Autodesk Fusion 360 part; units mm, degrees
(part 2 of 2)
extrude "Extrude27" add sketch "Back" against normal blind 3 separate body contours L0 L1 L2 L3 L6 L7 L8 L15 L16 L17 L20 L21 L22 L23 L24 L26 L29 L30 L31 L33 L34 L35 makes body 2
extrude "Extrude28" add sketch "Bottom" along normal blind 3 separate body contours L0 L1 L2 L3 L7 L8 L9 L11 L12 L13 L17 L19 L20 L23 L25 L26 L30 L31 L33 L34 L36 L37 L38 L39 L40 L44 L45 L47 makes body 3
combine "Combine15" operation cut target body 2 tool bodies 3 keep tools
combine "Combine16" operation cut target body 1 tool bodies 3 keep tools
extrude "Extrude29" add sketch "Right" against normal blind 3 separate body contours L0 L1 L2 L3 L7 L8 L9 L12 L13 L14 makes body 4
combine "Combine17" operation cut target body 4 tool bodies 1 keep tools
extrude "Extrude30" add sketch "Left" along normal blind 3 separate body contours L46 L47 L48 L49 L53 L54 L55 L57 L58 L59 makes body 5
combine "Combine18" operation cut target body 5 tool bodies 1 keep tools
combine "Combine19" operation cut target body 5 tool bodies 2 keep tools
combine "Combine20" operation cut target body 4 tool bodies 2 keep tools
combine "Combine21" operation cut target body 5 tool bodies 3 keep tools
combine "Combine22" operation cut target body 4 tool bodies 3 keep tools
combine "Combine23" operation cut target body 2 tool bodies 3 keep tools
extrude "Extrude31" add sketch "Top" against normal blind 3 separate body makes body 6
combine "Combine24" operation cut target body 6 tool bodies 5 keep tools
combine "Combine25" operation cut target body 6 tool bodies 1 keep tools
combine "Combine26" operation cut target body 6 tool bodies 4 keep tools
combine "Combine27" operation cut target body 6 tool bodies 2 keep tools
extrude "Extrude32" add sketch "BackSupport" along normal blind 3 separate body makes body 7
extrude "Extrude33" add sketch "FrontSupport" along normal blind 3 separate body makes body 8
combine "Combine28" operation cut target body 5 tool bodies 7 keep tools
combine "Combine29" operation cut target body 2 tool bodies 7 keep tools
combine "Combine30" operation cut target body 4 tool bodies 7 keep tools
combine "Combine31" operation cut target body 5 tool bodies 8 keep tools
combine "Combine32" operation cut target body 4 tool bodies 8 keep tools
extrude "Extrude11" [suppressed]
hidden bodies 6
equation "width = 57 mm"
equation "thick = 3 mm"
equation "d31 = -height / 2"
equation "d32 = width"
equation "d33 = length"
equation "d34 = finger"
equation "d35 = thick"
equation "d36 = finger"
equation "d37 = thick"
equation "d38 = finger"
equation "d39 = finger"
equation "d44 = length / 2"
equation "d45 = width"
equation "d46 = height"
equation "d47 = thick"
equation "d48 = finger"
equation "d49 = finger"
equation "height = 51.8 mm"
equation "length = 69 mm"
equation "finger = height / 5"
equation "d60 = -length / 2"
equation "d61 = width"
equation "d62 = height"
equation "d63 = thick"
equation "d64 = finger"
equation "d73 = width / 2"
equation "d74 = length"
equation "d75 = height"
equation "supportHeight = 22 mm + thick"
equation "d82 = -height / 2 + supportHeight"
equation "d83 = width / 2 - thick"
equation "d84 = length / 2 - thick"
equation "d85 = finger"
equation "d86 = backSupportWidth / 2"
equation "d87 = backSupportWidth / 2"
equation "d88 = thick"
equation "d89 = backSupportWidth / 2"
equation "d90 = thick"
equation "d91 = backSupportWidth / 2"
equation "backSupportDepth = 11 mm"
equation "backSupportCutout = 3 mm"
equation "d94 = backSupportWidth"
equation "d95 = backSupportDepth"
equation "d97 = width / 2 - thick - backSupportWidth"
equation "backSupportWidth = 8 mm"
equation "d102 = backSupportCutout"
equation "d103 = width / 2 - thick"
equation "d104 = length / 2 - thick"
equation "d105 = backSupportWidth / 2"
equation "d108 = backSupportWidth / 2"
equation "d109 = thick"
equation "d110 = backSupportWidth / 2"
equation "frontSupportDepth = 8 mm"
equation "d112 = backSupportWidth"
equation "d113 = frontSupportDepth"
equation "d114 = width / 2 - thick"
equation "d115 = length / 2 - thick"
equation "d117 = backSupportWidth"
equation "d118 = width / 2 - thick"
equation "d120 = width / 2 - backSupportWidth - thick"
equation "hexagonWidth = 6 mm"
equation "hexagonWall = 2 mm"
equation "d141 = thick"
equation "d242 = -width / 2"
equation "d243 = length / 2"
equation "d244 = height / 2"
equation "d245 = finger"
equation "d246 = thick + hexagonWall + hexagonWidth / 2"
equation "d247 = hexagonWidth / 2"
equation "d250 = hexagonWidth + hexagonWall"
equation "d254 = hexagonWidth + hexagonWall"
equation "d273 = thick"
equation "d277 = height / 2"
equation "d278 = width"
equation "d279 = length"
equation "d280 = finger"
equation "d281 = thick"
equation "d282 = finger"
equation "d283 = finger"
equation "d284 = thick"
equation "d285 = finger"
equation "d288 = finger"
equation "d289 = thick"
equation "d290 = finger"
equation "d291 = finger"
equation "d292 = thick"
equation "d293 = finger"
equation "d296 = length"
equation "d297 = height"
equation "d298 = finger"
equation "d299 = thick"
equation "d300 = finger"
equation "d301 = thick"
equation "d302 = finger"
equation "d303 = finger"
equation "d304 = thick"
equation "d306 = finger"
equation "d307 = thick"
equation "d308 = finger"
equation "d309 = thick"
equation "d310 = finger"
equation "d311 = finger"
equation "d314 = supportHeight - height / 2 + thick * 2 + 0.5 mm"
equation "d318 = width / 2"
equation "d319 = length / 2"
equation "d320 = width / 2"
equation "d321 = 23.5 mm + ( 13 / 2 ) * 1 mm"
equation "d326 = finger / 2"
equation "d327 = finger / 2"
equation "d329 = finger / 2"
equation "d330 = finger / 2"
equation "d332 = finger / 2"
equation "d333 = finger / 2"
equation "d334 = finger / 2"
equation "d335 = finger / 2"
equation "d368 = width / 2"
equation "d369 = height / 2"
equation "d370 = width / 2"
equation "d371 = thick + hexagonWall + hexagonWidth / 2"
equation "d372 = hexagonWidth / 2"
equation "d377 = length / 2"
equation "d378 = height / 2"
equation "d379 = finger"
equation "d380 = thick + hexagonWall + hexagonWidth / 2"
equation "d381 = hexagonWidth / 2"
equation "d398 = width / 2"
equation "d399 = length / 2"
equation "d400 = width / 2"
equation "d401 = hexagonWall + thick + hexagonWidth / 2"
equation "d402 = hexagonWidth / 2"
equation "d403 = thick"
equation "d405 = -thick"
equation "d407 = thick"
equation "d409 = -thick"
equation "d411 = thick"
equation "d413 = -thick"
equation "d415 = thick"
equation "d417 = thick"
named bodies: "Front", "Back", "Bottom", "Right", "Left", "Top", "BackSupport", "FrontSupport"
